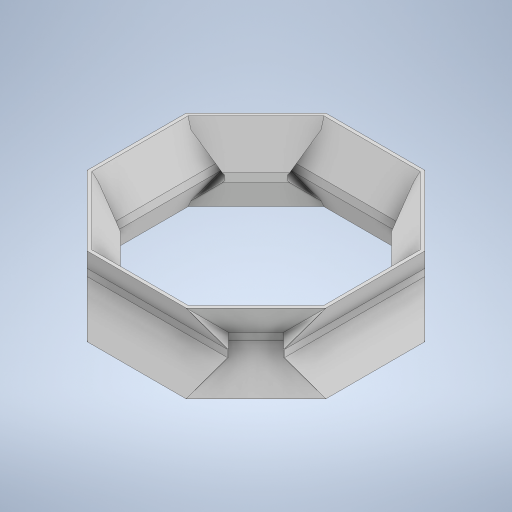
# Autodesk Inventor part: 팔각형 OV-PAM 층 한개
Saved by Autodesk Inventor 2024 (Build 280153000, 153)
## iProperties
Created: 2023-06-16
Part Number: 팔각형 OV-PAM 층 한개
Material: 일반
Document SubType Name: Modeling
Designer: jsw
Density: 1 g/cm^3
Appearance: 기본값
Mass: 4.59632 g
Surface Area: 118.739 cm^2
Volume: 4.59632 cm^3
Author: jsw
Autodesk Inventor part; units mm, degrees
ref_plane "YZ Plane" through (0, 0, 0) normal (1, 0, 0) x (0, 1, 0)
ref_plane "XZ Plane" through (0, 0, 0) normal (0, 1, 0) x (-1, 0, 0)
ref_plane "XY Plane" through (0, 0, 0) normal (0, 0, 1) x (1, 0, 0)
sketch "스케치1" plane through (0, 0, 0) normal (0, 1, 0) x (-1, 0, 0)
  line L0 (-32.5919, 13.5) -> (-13.5, 32.5919)
  line L1 (-13.5, 32.5919) -> (13.5, 32.5919)
  line L2 (13.5, 32.5919) -> (32.5919, 13.5)
  line L3 (32.5919, 13.5) -> (32.5919, -13.5)
  line L4 (32.5919, -13.5) -> (13.5, -32.5919)
  line L5 (13.5, -32.5919) -> (-13.5, -32.5919)
  line L6 (-13.5, -32.5919) -> (-32.5919, -13.5)
  line L7 (-32.5919, -13.5) -> (-32.5919, 13.5)
  line L8 (-13.8314, 33.3919) -> (13.8314, 33.3919)
  line L9 (13.8314, 33.3919) -> (33.3919, 13.8314)
  line L10 (33.3919, 13.8314) -> (33.3919, -13.8314)
  line L11 (33.3919, -13.8314) -> (13.8314, -33.3919)
  line L12 (13.8314, -33.3919) -> (-13.8314, -33.3919)
  line L13 (-13.8314, -33.3919) -> (-33.3919, -13.8314)
  line L14 (-33.3919, -13.8314) -> (-33.3919, 13.8314)
  line L15 (-33.3919, 13.8314) -> (-13.8314, 33.3919)
  point P0 (0, 0)
  point P1 (0, 0)
  point P2 (0, 0)
  dimension "d0" = 27
  dimension "d2" = 0.8
  constraints: 32 end point, 2 coincident, 2 horizontal, 34 other
  measures "d0" distance of L0.end L1.end
  measures "d2" distance between parallel lines of L10 L3
extrude "돌출2" add sketch "스케치1" along normal blind 10 contours L0 L1 L2 L3 L4 L5 L6 L7 | L8 L9 L10 L11 L12 L13 L14 L15
ref_plane "작업 평면2" through (33.3919, 0, 13.8314) normal (-0.8660254, -0.5, 0) x (0, 0, -1)
sketch "스케치3" plane through (33.3919, 0, 13.8314) normal (1, 0, 0) x (0, 0, -1)
  line L0 (0, 0) -> (0, 10) projected
  line L1 (0, 10) -> (27.6627, 10) projected
  line L2 (0, 0) -> (27.6627, 0)
  line L3 (27.6627, 0) -> (27.6627, 10)
  line L4 (27.6627, 10) -> (0, 10)
  line L5 (0, 10) -> (0, 0)
  line L6 (0, 10) -> (-5.9328, 10)
  line L7 (-19.5605, 10) -> (0, 10) projected
  line L8 (0, 0) -> (-5.9328, 10)
  line L9 (27.6627, 10) -> (33.5956, 10)
  line L10 (33.5956, 10) -> (27.6627, 0)
  point P0 (13.8314, 0)
  dimension "d17" = 120.68
  dimension "d18" = 120.68
  constraints: 16 end point, 2 parallel, 2 point on line, 1 horizontal, 1 perpendicular
  measures "d17" angle of L8 L2
  measures "d18" angle of L2 L10
extrude "돌출4" cut sketch "스케치3" against normal up to surface surface through (33.3919, 0, 13.8314) normal (-0.8660254, -0.5, 0)
sketch "스케치4" plane through (13.8314, 0, 33.3919) normal (0.7071068, 0, 0.7071068) x (0.7071068, 0, -0.7071068)
  line L0 (0, 0) -> (0, 10) projected
  line L1 (27.6627, 0) -> (27.6627, 10) projected
  line L2 (0, 0) -> (27.6627, 0)
  line L3 (27.6627, 0) -> (27.6627, 10)
  line L4 (27.6627, 10) -> (0, 10)
  line L5 (0, 10) -> (0, 0)
  line L6 (27.6627, 0) -> (19.4978, 10) projected
  line L7 (27.6627, 0) -> (19.2717, 10)
  line L8 (27.6627, 0) -> (0, 0) projected
  line L9 (0, 0) -> (8.391, 10)
  line L10 (27.6627, 10) -> (0, 10) projected
  point P0 (13.8314, 0)
  point P1 (8.391, 10)
  point P2 (27.6627, 0)
  dimension "d15" = 50
  dimension "d16" = 50
  constraints: 12 end point, 2 parallel, 2 point on line, 1 horizontal, 1 perpendicular
  measures "d15" angle of L7 L4
  measures "d16" angle of L4 L9
ref_plane "작업 평면3" through (13.8314, 0, 33.3919) normal (0.6123724, 0.5, 0.6123724) x (0.7071068, 0, -0.7071068)
extrude "돌출5" cut sketch "스케치4" against normal up to surface contours L9 L4 L7 L2 surface through (13.8314, 0, 33.3919) normal (0.6123724, 0.5, 0.6123724)
pattern_circular "원형 패턴1" count 4 over 360 about axis through (0, -10, 0) along (0, 1, 0) of "돌출4"
pattern_circular "원형 패턴2" count 4 over 360 about axis through (0, -10, 0) along (0, 1, 0) of "돌출5"
ref_plane "작업 평면4" through (0, 11, 0) normal (0, 1, 0) x (1, 0, 0)
sketch "스케치7" plane through (0, 11, 0) normal (0, 1, 0) x (1, 0, 0)
  line L0 (17.5239, -26.6946) -> (-17.5239, -26.6946) projected
  line L1 (-27.4586, -19.7647) -> (-23.3761, -15.6822) projected
  line L2 (-23.3761, -15.6822) -> (-15.6822, -23.3761) projected
  line L3 (-15.6822, -23.3761) -> (-19.7647, -27.4586) projected
  line L4 (-19.7647, -27.4586) -> (-19.6049, -27.6184) projected
  line L5 (-19.6049, -27.6184) -> (19.6049, -27.6184) projected
  line L6 (19.6049, -27.6184) -> (19.7647, -27.4586) projected
  line L7 (19.7647, -27.4586) -> (15.6822, -23.3761) projected
  line L8 (15.6822, -23.3761) -> (23.3761, -15.6822) projected
  line L9 (23.3761, -15.6822) -> (27.4586, -19.7647) projected
  line L10 (27.4586, -19.7647) -> (27.6184, -19.6049) projected
  line L11 (27.6184, -19.6049) -> (27.6184, 19.6049) projected
  line L12 (27.6184, 19.6049) -> (27.4586, 19.7647) projected
  line L13 (27.4586, 19.7647) -> (23.3761, 15.6822) projected
  line L14 (23.3761, 15.6822) -> (15.6822, 23.3761) projected
  line L15 (15.6822, 23.3761) -> (19.7647, 27.4586) projected
  line L16 (19.7647, 27.4586) -> (19.6049, 27.6184) projected
  line L17 (19.6049, 27.6184) -> (-19.6049, 27.6184) projected
  line L18 (-19.6049, 27.6184) -> (-19.7647, 27.4586) projected
  line L19 (-19.7647, 27.4586) -> (-15.6822, 23.3761) projected
  line L20 (-15.6822, 23.3761) -> (-23.3761, 15.6822) projected
  line L21 (-23.3761, 15.6822) -> (-27.4586, 19.7647) projected
  line L22 (-27.4586, 19.7647) -> (-27.6184, 19.6049) projected
  line L23 (-27.6184, 19.6049) -> (-27.6184, -19.6049) projected
  line L24 (-27.6184, -19.6049) -> (-27.4586, -19.7647) projected
  point P0 (0, 0)
extrude "돌출6" add sketch "스케치7" along normal mid plane 2
mirror "미러5" about plane through (0, 11, 0) normal (0, 1, 0) of "돌출2", "돌출5", "원형 패턴2", "돌출4", "원형 패턴1", "돌출6"
shell "쉘5" thickness 0.8 removed faces 2 at (11.1306, 22, 4.6105) at (4.6105, 0, -11.1306)
